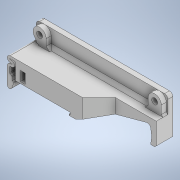
# Autodesk Inventor part: bracket_a
Saved by Autodesk Inventor 2020 (Build 240168000, 168)
## iProperties
Created: 2020-01-18
Part Number: bracket_a
Material: Generic
Document SubType Name: Modeling
Designer: yusaku
Density: 1 g/cm^3
Appearance: Default
Author: yusaku
Autodesk Inventor part; units mm, degrees
ref_plane "YZ Plane" through (0, 0, 0) normal (1, 0, 0) x (0, 1, 0)
ref_plane "XZ Plane" through (0, 0, 0) normal (0, 1, 0) x (-1, 0, 0)
sketch "Sketch1" plane through (0, 0, 0) normal (0, 0, 1) x (1, 0, 0)
  line L0 (-11.7, 0) -> (11.7, 0) construction
  arc A0 (11.7, 0) -> (13.5, 1.8) centre (11.7, 1.8) ccw construction
  line L1 (13.5, 1.8) -> (13.5, 5.7) construction
  arc A1 (14.3, 6.5) -> (13.5, 5.7) centre (14.3, 5.7) ccw construction
  line L2 (14.3, 6.5) -> (17.5, 6.5) construction
  line L3 (17.5, 6.5) -> (17.5, 7.5) construction
  line L4 (17.5, 7.5) -> (14.3, 7.5) construction
  arc A2 (14.3, 7.5) -> (12.5, 5.7) centre (14.3, 5.7) ccw construction
  line L5 (12.5, 5.7) -> (12.5, 1.8) construction
  arc A3 (11.7, 1) -> (12.5, 1.8) centre (11.7, 1.8) ccw construction
  line L6 (11.7, 1) -> (-11.7, 1) construction
  arc A4 (-12.5, 1.8) -> (-11.7, 1) centre (-11.7, 1.8) ccw construction
  line L7 (-12.5, 1.8) -> (-12.5, 5.7) construction
  arc A5 (-12.5, 5.7) -> (-14.3, 7.5) centre (-14.3, 5.7) ccw construction
  line L8 (-14.3, 7.5) -> (-17.5, 7.5) construction
  line L9 (-17.5, 7.5) -> (-17.5, 6.5) construction
  line L10 (-17.5, 6.5) -> (-14.3, 6.5) construction
  arc A6 (-13.5, 5.7) -> (-14.3, 6.5) centre (-14.3, 5.7) ccw construction
  line L11 (-13.5, 5.7) -> (-13.5, 1.8) construction
  arc A7 (-13.5, 1.8) -> (-11.7, 0) centre (-11.7, 1.8) ccw construction
  line L12 (-18.95, 19) -> (25, 19)
  line L13 (25, 19) -> (25, 7.5)
  line L14 (25, 7.5) -> (-15.7, 7.5)
  line L15 (17.7, 7.5) -> (17.7, 6.5)
  line L16 (17.7, 6.5) -> (17, 6.3124)
  line L17 (17, 6.3124) -> (17, 5.5)
  line L18 (17, 5.5) -> (20.7426, 5.5)
  line L19 (20.7426, 5.5) -> (25, 7.5)
  line L20 (-17.7, 8.5566) -> (-17.7, 6.5)
  line L21 (-17.7, 6.5) -> (-16.7, 6.2321)
  line L22 (-16.7, 5.8321) -> (-17.9306, 2.451)
  arc A8 (-20.7, 2.9393) -> (-17.9306, 2.451) centre (-19.2723, 2.9393) ccw
  line L23 (-20.7, 2.9393) -> (-20.7, 13)
  line L24 (-15.7, 7.5) -> (-15.7, 17)
  line L25 (-20, 20) -> (60, 20)
  line L26 (60, 20) -> (60, 29)
  line L27 (60, 29) -> (-20, 29)
  line L28 (-20, 29) -> (-20, 20)
  line L29 (60, 19) -> (60, 20)
  line L30 (25, 7.5) -> (60, 17)
  line L31 (-16.7, 6.2321) -> (-16.7, 5.8321)
  line L32 (-19.2, 10) -> (-8.8081, 10) construction
  line L33 (-8.8081, 10) -> (-8.8081, 13) construction
  line L34 (-8.8081, 13) -> (-19.2, 13) construction
  arc A9 (-18.95, 19) -> (-18.95, 15.5) centre (-18.95, 17.25) ccw
  arc A10 (-18.95, 17.5) -> (-18.95, 17) centre (-18.95, 17.25) ccw
  line L35 (-18.95, 17.5) -> (-16.2, 17.5)
  arc A11 (-15.7, 17) -> (-16.2, 17.5) centre (-16.2, 17) ccw
  arc A12 (-15.7, 19) -> (-16.7, 20) centre (-16.7, 19) ccw
  line L36 (25, 19) -> (60, 19)
  circle A13 centre (-15, 25) radius 4 construction
  line L37 (60, 17) -> (60, 19)
  line L38 (60, 17) -> (60, 5)
  line L39 (60, 5) -> (56.7, 5)
  line L40 (56.7, 5) -> (56.7, 6)
  arc A14 (56.7, 6) -> (56.7, 12.9022) centre (37, 9.4511) ccw
  line L41 (56.7, 12.9022) -> (56.1645, 15.9589)
  arc A15 (56.5428, 13.7996) -> (54.0489, 15.3847) centre (54.5728, 13.4545) ccw
  line L42 (57, 5) -> (57, 16.1857) construction
  line L43 (-19.2, 10) -> (-19.2, 13)
  arc A16 (-18.7, 13.5) -> (-19.2, 13) centre (-18.7, 13) ccw
  arc A17 (-19.2, 10) -> (-18.95, 9.567) centre (-18.7, 10) ccw
  line L44 (-18.95, 9.567) -> (-17.95, 8.9896)
  arc A18 (-17.7, 8.5566) -> (-17.95, 8.9896) centre (-18.2, 8.5566) ccw
  arc A19 (-18.7, 15) -> (-20.7, 13) centre (-18.7, 13) ccw
  line L45 (-18.95, 17) -> (-18, 17)
  line L46 (-18.95, 15.5) -> (-18, 15.5)
  line L47 (-20.7, 13) -> (-20.7, 17.25) construction
  arc A20 (-18, 13.5) -> (-18, 17) centre (-18, 15.25) ccw
  arc A21 (-18, 15) -> (-18, 15.5) centre (-18, 15.25) ccw
  line L48 (-18.7, 13.5) -> (-18, 13.5)
  line L49 (-18, 15) -> (-18.7, 15)
  point P0 (0, 0)
  point P1 (0, 0)
  point P2 (25.6678, 15)
  point P3 (25.6678, 15)
  point P4 (-16.7, 6.0321)
  point P5 (56.4632, 14.0537)
  dimension "d0" = 35
  dimension "d1" = 25
  dimension "d2" = 1
  dimension "d3" = 0.8
  dimension "d4" = 7.5
  dimension "d6" = 0.2
  dimension "d10" = 3
  dimension "d11" = 3.5607
  dimension "d12" = 0.2
  dimension "d16" = 11.5
  dimension "d24" = 2
  dimension "d26" = 80
  dimension "d27" = 9
  dimension "d30" = 20
  dimension "d40" = 20
  dimension "d41" = 1
  dimension "d43" = 75
  dimension "d44" = 1
  dimension "d48" = 3
  dimension "d49" = 2.5
  dimension "d50" = 0.5
  dimension "d59" = 8
  dimension "d60" = 15
  dimension "d61" = 25
  dimension "d66" = 2
  dimension "d67" = 2
  dimension "d97" = 0.4
  dimension "d98" = 0.7
  dimension "d99" = 20
  dimension "d100" = 0.8124
  dimension "d101" = 1
  dimension "d102" = 75
  dimension "d105" = 25
  dimension "d109" = 1
  dimension "d110" = 3.3
  dimension "d111" = 2
  dimension "d112" = 20
  dimension "d113" = 3
  dimension "d120" = 5
  dimension "d133" = 1.75
  dimension "d134" = 1.5
  dimension "d136" = 60
  dimension "d137" = 0.5
  dimension "d138" = 1.5
  dimension "d146" = 0.25
  dimension "d147" = 2.7
  constraints: 103 end point, 43 point on circle, 40 tangent, 22 centre point, 16 perpendicular, 12 point on line, 9 horizontal, 9 vertical, 7 concentric, 7 parallel, 6 equal radius, 3 collinear, 2 midpoint, 1 coincident, 1 line through centre, 1 vertical alignment
  measures "d0" distance between parallel lines of L3 L9
  measures "d1" distance between parallel lines of L5 L7
  measures "d2" distance of L8.end L9.end
  measures "d3" radius of A6
  measures "d4" distance between parallel lines of L4 L0
  measures "d6" distance between parallel lines of L15 L3
  measures "d10" distance between parallel lines of L23 L20
  measures "d11" vertical distance of A8.centre L20.end
  measures "d12" distance between parallel lines of L20 L9
  measures "d16" distance of L12.end L13.end
  measures "d24" distance between parallel lines of L20 L24
  measures "d26" distance of L27.end L26.end
  measures "d27" distance of L26.end L25.end
  measures "d30" distance from line of L28 point (0, 0)
  measures "d40" distance between parallel lines of L0 L25
  measures "d41" distance between parallel lines of L25 L12
  measures "d43" angle of L20 L21
  measures "d44" distance from line of L20 L21.end
  measures "d48" distance of L32.end L33.end
  measures "d49" distance between parallel lines of L14 L32
  measures "d50" radius of A11
  measures "d59" diameter of A13
  measures "d60" horizontal distance of point (0, 0) A13.centre
  measures "d61" distance from line of A13.centre L0
  measures "d66" distance of L30.end L29.start
  measures "d67" distance between parallel lines of L14 L18
  measures "d97" distance of L21.end L22.start
  measures "d98" distance between parallel lines of L15 L17
  measures "d99" angle of L31 L22
  measures "d100" distance of L16.end L17.end
  measures "d101" distance of L15.start L15.end
  measures "d102" angle of L15 L16
  measures "d105" distance from line of point (0, 0) L13
  measures "d109" distance of L39.end L40.end
  measures "d110" distance of L38.end L39.end
  measures "d111" radius of A15
  measures "d112" radius of A14
  measures "d113" distance between parallel lines of L38 L42
  measures "d120" distance between parallel lines of L39 L0
  measures "d133" radius of A9
  measures "d134" distance between parallel lines of L12 L35
  measures "d136" angle of L20 L44
  measures "d137" radius of A17
  measures "d138" distance between parallel lines of L23 L43
  measures "d146" radius of A10
  measures "d147" distance from line of L47 A20.centre
extrude "Extrusion1" add sketch "Sketch1" along normal blind 10 contours L12 L13 L14 L24 A11 L35 A10 L45 A20 L48 A16 L43 A17 L44 A18 L20 L21 L31 L22 A8 L23 A19 L49 A21 L46 A9 | L36 L37 L30 L13 | L19 L18 L17 L16 L15 L14 | L30 L41 A15 | L38 L39 L40 A14 L41 L30
sketch "Sketch6" plane through (0, 0, 10) normal (0, 0, 1) x (1, 0, 0)
  line L0 (20.7426, 5.5) -> (25, 7.5) projected
  line L1 (25, 7.5) -> (54.0489, 15.3847) projected
  arc A0 (56.5428, 13.7996) -> (54.0489, 15.3847) centre (54.5728, 13.4545) ccw projected
  line L2 (56.5428, 13.7996) -> (56.7, 12.9022) projected
  arc A1 (56.7, 6) -> (56.7, 12.9022) centre (37, 9.4511) ccw projected
  line L3 (56.7, 6) -> (56.7, 5) projected
  line L4 (56.7, 5) -> (60, 5) projected
  line L5 (60, 5) -> (60, 19) projected
  line L6 (60, 19) -> (-18.95, 19) projected
  arc A2 (-18.95, 19) -> (-18.95, 15.5) centre (-18.95, 17.25) ccw projected
  line L7 (-20.7, 13) -> (-20.7, 2.9393) projected
  arc A3 (-20.7, 2.9393) -> (-17.9306, 2.451) centre (-19.2723, 2.9393) ccw projected
  line L8 (-17.9306, 2.451) -> (-16.7, 5.8321) projected
  line L9 (-16.7, 5.8321) -> (-16.7, 6.2321) projected
  line L10 (-16.7, 6.2321) -> (-17.7, 6.5) projected
  line L11 (-17.7, 6.5) -> (-17.7, 8.5566) projected
  arc A4 (-18.95, 17.5) -> (-18.95, 17) centre (-18.95, 17.25) ccw projected
  line L12 (-18.95, 17.5) -> (-16.2, 17.5) projected
  arc A5 (-15.7, 17) -> (-16.2, 17.5) centre (-16.2, 17) ccw projected
  line L13 (-15.7, 17) -> (-15.7, 7.5) projected
  line L14 (-15.7, 7.5) -> (17.7, 7.5) projected
  line L15 (17.7, 7.5) -> (17.7, 6.5) projected
  line L16 (17.7, 6.5) -> (17, 6.3124) projected
  line L17 (17, 6.3124) -> (17, 5.5) projected
  line L18 (17, 5.5) -> (20.7426, 5.5) projected
  line L19 (20.7426, 5.5) -> (25, 7.5) projected
  line L20 (25, 7.5) -> (25, 19)
  line L21 (-18.95, 15.5) -> (-18, 15.5) projected
  arc A6 (-18, 15) -> (-18, 15.5) centre (-18, 15.25) ccw projected
  line L22 (-18, 15) -> (-18.7, 15) projected
  arc A7 (-18.7, 15) -> (-20.7, 13) centre (-18.7, 13) ccw projected
  arc A8 (-17.7, 8.5566) -> (-17.95, 8.9896) centre (-18.2, 8.5566) ccw projected
  line L23 (-17.95, 8.9896) -> (-18.95, 9.567) projected
  arc A9 (-19.2, 10) -> (-18.95, 9.567) centre (-18.7, 10) ccw projected
  line L24 (-19.2, 10) -> (-19.2, 13) projected
  arc A10 (-18.7, 13.5) -> (-19.2, 13) centre (-18.7, 13) ccw projected
  line L25 (-18.7, 13.5) -> (-18, 13.5) projected
  arc A11 (-18, 13.5) -> (-18, 17) centre (-18, 15.25) ccw projected
  line L26 (-18, 17) -> (-18.95, 17) projected
  point P0 (0, 0)
  constraints: 2 end point, 1 perpendicular, 1 point on line
extrude "Extrusion5" add sketch "Sketch6" along normal blind 10 contours L18 L17 L16 L15 L14 L13 A5 L12 A4 L26 A11 L25 A10 L24 A9 L23 A8 L11 L10 L9 L8 A3 L7 A7 L22 A6 L21 A2 L6 L20 L0
extrude "Extrusion2" add sketch "Sketch1" along normal blind 3 contours A12 L25 L29 L36 L12 | L25 L28 L27 L26
sketch "Sketch2" plane through (0, 0, 3) normal (0, 0, 1) x (1, 0, 0)
  line L0 (-11, 25) -> (-11, 19)
  line L1 (-20, 29) -> (-20, 20) projected
  arc A0 (-11, 25) -> (-17.9751, 22.3262) centre (-15, 25) ccw
  line L2 (60, 29) -> (-20, 29) projected
  line L3 (-20, 20) -> (-16.7, 20) projected
  arc A1 (-15.7, 19) -> (-16.7, 20) centre (-16.7, 19) ccw projected
  arc A2 (-16.7, 19) -> (-17.9751, 22.3262) centre (-21.6761, 19) ccw
  arc A3 (59, 25) -> (51, 25) centre (55, 25) ccw
  line L4 (51, 25) -> (51, 19)
  line L5 (59, 25) -> (59, 19)
  line L6 (60, 19) -> (-15.7, 19) projected
  point P0 (0, 0)
  point P1 (-15, 29)
  point P2 (-16.8015, 20)
  dimension "d56" = 25
  dimension "d57" = 15
  dimension "d58" = 4
  dimension "d62" = 4
  dimension "d63" = 55
  constraints: 6 end point, 6 point on circle, 4 tangent, 3 centre point, 2 perpendicular, 1 horizontal alignment, 1 line through centre, 1 vertical
  measures "d56" vertical distance of point (0, 0) A0.centre
  measures "d57" horizontal distance of point (0, 0) A0.centre
  measures "d58" radius of A0
  measures "d62" radius of A3
  measures "d63" horizontal distance of point (0, 0) A3.centre
extrude "Extrusion3" add sketch "Sketch2" along normal blind 3 contours L0 L6 A1 L3 A2 A0 | L4 A3 L5 L6
chamfer "Chamfer1" distance 2 angle 45 3 edges at (-11, 19, 4.5) (20, 19, 3) (51, 19, 4.5)
chamfer "Chamfer2" distance 1 angle 45 2 edges at (59, 19, 4.5) (60, 5, 5)
fillet "Fillet1" radius 2 3 edges at (60, 29, 1.5) (-20, 29, 1.5) (-20, 20, 1.5)
sketch "Sketch3" plane through (0, 0, 6) normal (0, 0, 1) x (1, 0, 0)
  arc A0 (59, 25) -> (51, 25) centre (55, 25) ccw projected
  arc A1 (-11, 25) -> (-17.9751, 22.3262) centre (-15, 25) ccw projected
  point P0 (0, 0)
  constraints: 2 coincident
hole "Hole1" at (55, 25, 6) at (-15, 25, 6) direction (0, 0, -1) diameter 3.6 end through all
sketch "Sketch4" plane through (-20.7, 5.1959, 0) normal (-1, 0, 0) x (0, 0, 1)
  line L0 (8.4123, 3.5541) -> (6.8246, 6.3041)
  line L1 (6.8246, 6.3041) -> (8.4123, 9.0541)
  line L2 (8.4123, 9.0541) -> (11.5877, 9.0541)
  line L3 (11.5877, 9.0541) -> (13.1754, 6.3041)
  line L4 (13.1754, 6.3041) -> (11.5877, 3.5541)
  line L5 (11.5877, 3.5541) -> (8.4123, 3.5541)
  line L6 (0, 2.3041) -> (10, 2.3041) projected
  line L7 (0, 13.8041) -> (20, 13.8041) projected
  line L8 (10, 13.8041) -> (10, 2.3041) construction
  line L9 (0, 2.3041) -> (20, 2.3041) projected
  line L10 (0, 2.3041) -> (20, 2.3041) projected
  point P0 (0, -5.1959)
  point P1 (10, 6.3041)
  point P2 (10, 8.0541)
  dimension "d82" = 5.5
  dimension "d83" = 10
  dimension "d148" = 4
  constraints: 14 end point, 2 midpoint, 1 horizontal, 1 point on line, 1 vertical, 13 other
  measures "d82" distance between parallel lines of L5 L2
  measures "d83" horizontal distance of point (0, -5.196) point (10, 6.304)
  measures "d148" distance from line of L9 point (10, 6.304)
hole "Hole2" at (-20.7, 11.5, 10) direction (1, 0, 0) diameter 3.5 depth 20
ref_plane "Work Plane1" through (-12.7, 7.5, 0) normal (-1, 0, 0) x (0, 0, 1)
sketch "Sketch5" plane through (-12.7, 7.5, 0) normal (-1, 0, 0) x (0, 0, 1)
  line L0 (8.1813, 0.85) -> (6.3627, 4)
  line L1 (6.3627, 4) -> (8.1813, 7.15)
  line L2 (8.1813, 7.15) -> (11.8187, 7.15)
  line L3 (11.8187, 7.15) -> (13.6373, 4)
  line L4 (13.6373, 4) -> (11.8187, 0.85)
  line L5 (11.8187, 0.85) -> (8.1813, 0.85)
  circle A0 centre (10, 4) radius 1.75 construction
  line L6 (11.9341, 1.05) -> (25, 1.05)
  line L7 (25, 1.05) -> (25, 6.95)
  line L8 (25, 6.95) -> (11.9341, 6.95)
  line L9 (10, 0) -> (10, 7.8847) projected
  line L10 (10, 7.8847) -> (10, 6.2996) projected
  line L11 (10, 5.4022) -> (10, -1.5) projected
  line L12 (10, -1.5) -> (10, -2.5) projected
  line L13 (10, -1.5) -> (10, 11.5) projected
  line L14 (10, -1.5) -> (10, -2.5) projected
  line L15 (10, 6.2996) -> (10, 5.4022) projected
  line L16 (10, 11.5) -> (10, 0) projected
  line L17 (20, 0) -> (20, 11.5) projected
  point P0 (0, -7.5)
  point P1 (25, 4)
  dimension "d92" = 6.3
  dimension "d95" = 5.9
  dimension "d116" = 5
  constraints: 18 end point, 2 horizontal, 2 point on line, 1 coincident, 1 horizontal alignment, 1 midpoint, 1 perpendicular, 13 other
  measures "d92" distance between parallel lines of L5 L2
  measures "d95" distance between parallel lines of L8 L6
  measures "d116" distance between parallel lines of L7 L17
extrude "Extrusion4" cut sketch "Sketch5" against normal blind 3
chamfer "Chamfer3" distance 10 angle 45 1 edges at (25, 13.25, 10)
sketch "スケッチ7" plane through (0, 0, 0) normal (0, 0, -1) x (-1, 0, 0)
  line L0 (-53.3546, 27.85) -> (-51.7091, 25)
  line L1 (-51.7091, 25) -> (-53.3546, 22.15)
  line L2 (-53.3546, 22.15) -> (-56.6454, 22.15) construction
  line L3 (-56.6454, 22.15) -> (-58.2909, 25) construction
  line L4 (-58.2909, 25) -> (-56.6454, 27.85)
  line L5 (-56.6454, 27.85) -> (-53.3546, 27.85)
  circle A0 centre (-55, 25) radius 1.8 projected
  line L6 (-53.6876, 28.2732) -> (-53.9319, 27.85)
  line L7 (-53.9319, 27.85) -> (-53.0659, 27.35) construction
  line L8 (-53.0659, 27.35) -> (-52.8215, 27.7732)
  line L9 (-52.8215, 27.7732) -> (-53.6876, 28.2732)
  line L10 (-53.2546, 28.0232) -> (-53.4989, 27.6) construction
  line L11 (-55, 27.85) -> (-55, 25)
  line L12 (-55, 25) -> (-52.5318, 26.425)
  line L13 (-52.9504, 27.55) -> (-53.2081, 27.9964)
  line L14 (-53.8164, 28.05) -> (-53.301, 28.05)
  point P0 (0, 0)
  point P1 (-53.4412, 25.9)
  point P2 (-55, 26.8)
  dimension "d121" = 5.7
  dimension "d124" = 1
  dimension "d125" = 0.2
  dimension "d132" = 0.2
  constraints: 30 end point, 7 point on line, 4 midpoint, 4 parallel, 1 coincident, 1 equal length, 1 horizontal, 1 perpendicular, 1 vertical, 13 other
  measures "d121" distance between parallel lines of L2 L5
  measures "d124" distance of L8.end L6.start
  measures "d125" distance from line of L9 L0.start
  measures "d132" distance between parallel lines of L0 L13
extrude "押し出し6" cut sketch "スケッチ7" against normal blind 2.5 contours L5 L6 L14 L9 L13 L8 L0 | L0 L12 A0 L11 L5
pattern_circular "円形状パターン1" count 6 over 360 about axis through (55, 25, -81.5677) along (0, 0, 1) of "押し出し6"
pattern_linear "矩形状パターン1" count 2 spacing 70 along (-1, 0, 0) of "押し出し6", "円形状パターン1"
body "Solid1"
